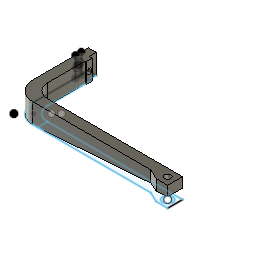
Voron2 Camera Mount (Autodesk Fusion 360 design; units mm, degrees)
Autodesk Fusion 360 part; units mm, degrees
sketch "Sketch1" plane through (0, 0, 0) normal (0, 0, 1) x (1, 0, 0)
  line L0 (0, 19) -> (0, 75)
  line L1 (0, 75) -> (8, 75)
  line L2 (10, 68) -> (10, 24)
  line L3 (24, 10) -> (160, 10)
  line L4 (10, 68) -> (8, 68)
  line L5 (8, 68) -> (8, 75)
  arc A0 (0, 19) -> (19, 0) centre (19, 19) ccw
  arc A1 (10, 24) -> (24, 10) centre (24, 24) ccw
  circle A2 centre (152.5, 2.5) radius 3.175
  circle A3 centre (152.5, 2.5) radius 5
  line L6 (160, -5) -> (148.2812, -5)
  line L7 (148.2812, -5) -> (138, 0)
  line L8 (19, 0) -> (138, 0)
  line L9 (160, 10) -> (160, -5)
  line L10 (24, 10) -> (24, 0)
  point P0 (10, 10)
  dimension "d1" = 7
  dimension "d2" = 75
  dimension "d5" = 19
  dimension "d6" = 14
  dimension "d13" = 6.35
  dimension "d14" = 10
  dimension "d18" = 7.5
  dimension "d19" = 15
  dimension "d20" = 119
  dimension "d42" = 7.5
  dimension "d43" = 160
  constraint vertical L0
  constraint perpendicular L0 L1
  constraint perpendicular L1 L2
  constraint perpendicular L0 L3
  constraint perpendicular L2 L4
  constraint perpendicular L1 L5
  constraint coincident origin L0
  constraint coincident origin L8
  constraint tangent L0 A0
  constraint tangent A0 L8
  constraint coincident P0 L2
  constraint coincident P0 L3
  constraint tangent L2 A1
  constraint tangent L3 A1
  constraint concentric A2 A3
  constraint perpendicular L6 L9
  constraint coincident L8 L10.end
  constraint perpendicular L8 L10
  measures "d1" distance of L4.end L1.end
  measures "d2" distance of origin L0.end
  measures "d5" radius of A0
  measures "d6" radius of A1
  measures "d13" diameter of A2
  measures "d14" diameter of A3
  measures "d18" distance of A2.centre L6
  measures "d19" distance of L3 L6
  measures "d20" distance of A0.end L7.end
  measures "d42" distance of A2.centre L9
  measures "d43" distance of L0 L9
extrude "Extrude1" add sketch "Sketch1" along normal blind 20 contours L0 L1 L2 L4 L5 A0 A1 L8 L10 | L3 L6 L7 L8 L9 L10 | A3
extrude "Extrude3" cut sketch "Sketch1" along normal blind 15 contours A3
sketch "Sketch2" plane through (0, 0, 0) normal (-1, 0, 0) x (0, -1, 0)
  line L0 (-75, 0) -> (-19, 0)
  line L1 (-19, 0) -> (-19, 20)
  line L2 (-19, 20) -> (-75, 20)
  line L3 (-75, 20) -> (-75, 0)
  circle A0 centre (-65, 10) radius 2.6
  circle A1 centre (-65, 10) radius 5
  line L4 (-68, 20) -> (-68, 0)
  line L5 (-62, 20) -> (-62, 0)
  dimension "d23" = 5.2
  dimension "d24" = 10
  dimension "d25" = 10
  dimension "d26" = 10
  dimension "d31" = 20
  dimension "d32" = 20
  dimension "d33" = 7
  dimension "d34" = 13
  constraint concentric A0 A1
  constraint coincident L2 L4.start
  constraint vertical L4
  constraint coincident L2 L5.start
  constraint vertical L5
  measures "d23" diameter of A0
  measures "d24" diameter of A1
  measures "d25" distance of L3 A0.centre
  measures "d26" distance of L2 A0.centre
  measures "d31" distance of L4.start L4.end
  measures "d32" distance of L5.start L5.end
  measures "d33" distance of L3 L4
  measures "d34" distance of L3 L5
extrude "Extrude4" cut sketch "Sketch2" against normal blind 10 contours A0
extrude "Extrude5" cut sketch "Sketch2" against normal blind 7 contours A1 L4 L5 | A1 L4 | A1 L5
extrude "Extrude6" add sketch "Sketch2" against normal blind 1 from surface at -10 contours L0 A1 L4 L5 | A1 L4 L5 | L2 A1 L4 L5
sketch "Sketch5" plane through (0, 10, 0) normal (0, 1, 0) x (-1, 0, 0)
  line L0 (-160, 0) -> (-24, 0)
  line L1 (-24, 0) -> (-24, 20)
  line L2 (-24, 20) -> (-160, 20)
  line L3 (-160, 20) -> (-160, 0)
  line L4 (-24, 0) -> (-160, 10)
  constraint coincident L0.end L1.start
  constraint midpoint L3 L4.end
extrude "Extrude8" cut sketch "Sketch5" against normal blind 15 contours L0 L3 L4
equation "d20 = 69 mm + 50 mm"
